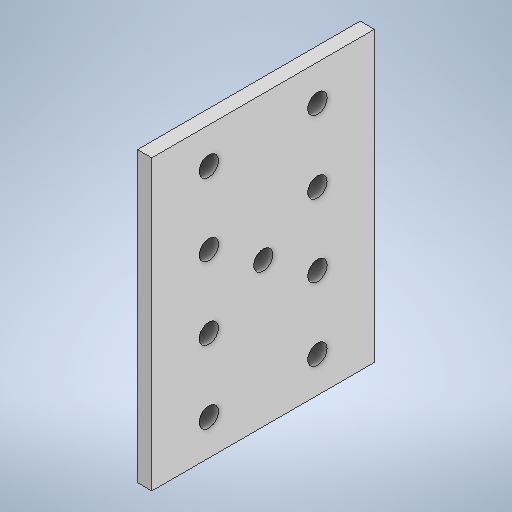
# Autodesk Inventor part: base_plate
Saved by Autodesk Inventor 2025 (Build 290162000, 162)
## iProperties
Created: 2025-12-10
Part Number: base_plate
Material: Generic
Document SubType Name: Modeling
Designer: GOLZARDM
Density: 1 g/cm^3
Appearance: Default
Author: GOLZARDM
Autodesk Inventor part; units mm, degrees
ref_plane "YZ Plane" through (0, 0, 0) normal (1, 0, 0) x (0, 1, 0)
ref_plane "XZ Plane" through (0, 0, 0) normal (0, 1, 0) x (-1, 0, 0)
ref_plane "XY Plane" through (0, 0, 0) normal (0, 0, 1) x (1, 0, 0)
sketch "Sketch5" plane through (0, 0, 0) normal (1, 0, 0) x (0, 1, 0)
  line L0 (50.6, -39.05) -> (-50.6, -39.05)
  line L1 (-50.6, -39.05) -> (-50.6, 39.05)
  line L2 (-50.6, 39.05) -> (50.6, 39.05)
  line L3 (50.6, 39.05) -> (50.6, -39.05)
  line L4 (50.6, -39.05) -> (-50.6, 39.05) construction
  line L5 (-50.6, -39.05) -> (50.6, 39.05) construction
  point P0 (0, 0)
  dimension "d31" = 78.1
  dimension "d32" = 101.2
  constraints: 12 end point, 2 midpoint, 2 parallel, 1 horizontal, 1 perpendicular
  measures "d31" distance of L2.end L0.start
  measures "d32" distance of L0.start L0.end
extrude "Extrusion2" add sketch "Sketch5" along normal blind 5
sketch "Sketch10" plane through (5, 0, 0) normal (1, 0, 0) x (0, 0, -1)
  line L0 (39.05, 50.6) -> (-39.05, 50.6) projected
  line L1 (39.05, -50.6) -> (39.05, 50.6) projected
  point P0 (0, 0)
  point P1 (19.05, 38.1)
  dimension "d93" = 12.5
  dimension "d103" = 20
  measures "d93" distance from line of L0 point (19.05, 38.1)
  measures "d103" distance from line of L1 point (19.05, 38.1)
hole "Hole8" at (5, 38.1, -19.05) direction (-1, 0, 0) diameter 6.8 end through all
sketch "Sketch11" plane through (5, 0, 0) normal (1, 0, 0) x (0, 0, -1)
  circle A0 centre (19.05, 38.1) radius 3.4 projected
  point P0 (0, 0)
  point P1 (-19.05, 38.1)
  dimension "d85" = 38.1
  dimension "d86" = 0
  measures "d85" distance of A0.centre point (-19.05, 38.1)
  measures "d86" vertical distance of point (-19.05, 38.1) A0.centre
hole "Hole9" at (5, 38.1, 19.05) direction (-1, 0, 0) diameter 6.8 end through all
pattern_linear "Rectangular Pattern1" count 6 spacing 25.4 along (0, -1, 0) of "Hole8"
pattern_linear "Rectangular Pattern2" count 6 spacing 25.4 along (0, -1, 0) of "Hole9"
sketch "Sketch12" plane through (5, 0, 0) normal (1, 0, 0) x (0, 0, -1)
  line L0 (39.05, -50.6) -> (39.05, 50.6) projected
  line L1 (-39.05, -50.6) -> (39.05, -50.6) projected
  point P0 (0, 0)
  point P1 (0.04, 0)
  dimension "d101" = 39.01
  dimension "d102" = 50.6
  measures "d101" distance from line of L0 point (0.04, 0)
  measures "d102" distance from line of L1 point (0.04, 0)
hole "Hole10" at (5, 0, -0.04) direction (-1, 0, 0) diameter 6.75 end through all
body "Solid2"
